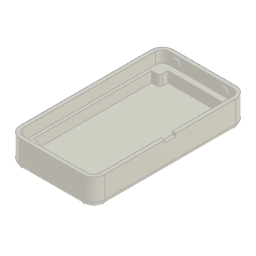
NodeMCU_Case_v9 (Autodesk Fusion 360 design; units mm, degrees)
Autodesk Fusion 360 part; units mm, degrees
note: some values were not read from the file. Set by a fixed rule: which sketch regions a step uses.
sketch "Skizze1" plane through (0, 0, 0) normal (0, 0, 1) x (1, 0, 0)
  line L0 (-15.4, 27.9) -> (15.4, 27.9)
  line L1 (15.4, 27.9) -> (15.4, -27.9)
  line L2 (15.4, -27.9) -> (-15.4, -27.9)
  line L3 (-15.4, -27.9) -> (-15.4, 27.9)
  line L4 (0, 70) -> (0, 58.2849) construction
  line L5 (30, 0) -> (40, 0) construction
  line L6 (-13.8, 26.3) -> (13.8, 26.3)
  line L7 (13.8, 26.3) -> (13.8, -26.3)
  line L8 (13.8, -26.3) -> (-13.8, -26.3)
  line L9 (-13.8, -26.3) -> (-13.8, 26.3)
  line L10 (-13, 24.5) -> (13, 24.5)
  line L11 (13, 24.5) -> (13, -24.5)
  line L12 (13, -24.5) -> (-13, -24.5)
  line L13 (-13, -24.5) -> (-13, 24.5)
  line L14 (-13, 19.5) -> (-10.03, 19.5)
  line L15 (-10.03, 19.5) -> (-10.03, -19.4987)
  line L16 (10.03, 19.5) -> (10.03, -19.4987)
  line L17 (13, 19.5) -> (10.03, 19.5)
  line L18 (-10.03, -19.4987) -> (-13, -19.4987)
  line L19 (10.03, -19.4987) -> (13, -19.4987)
  circle A0 centre (10.5, 21.7) radius 1.5
  circle A1 centre (-10.5, 21.7) radius 1.5
  circle A2 centre (10.5, -21.7) radius 1.5
  circle A3 centre (-10.5, -21.7) radius 1.5
  line L20 (-7.03, 20) -> (-7.03, -20)
  spline S0 degree 5 poles (-7.03, 20) (-6.9803, 20.007) (-6.8827, 20.0236) (-6.7413, 20.0561) (-6.5626, 20.1135) (-6.3549, 20.2028) (-6.1611, 20.3033) (-5.9792, 20.41) (-5.8066, 20.5219) (-5.6404, 20.6442) (-5.4777, 20.7847) (-5.3165, 20.9514) (-5.1557, 21.1497) (-4.9962, 21.3794) (-4.8409, 21.6328) (-4.6934, 21.8985) (-4.5577, 22.1636) (-4.4367, 22.4166) (-4.3316, 22.6498) (-4.2411, 22.8631) (-4.161, 23.0622) (-4.0871, 23.256) (-4.0155, 23.4531) (-3.9446, 23.6591) (-3.8764, 23.8734) (-3.816, 24.0904) (-3.7783, 24.2602) (-3.7581, 24.3824) (-3.7486, 24.4613) (-3.7448, 24.5) knots 0 0 0 0 0 0 0.04 0.08 0.12 0.16 0.2 0.24 0.28 0.32 0.36 0.4 0.44 0.48 0.52 0.56 0.6 0.64 0.68 0.72 0.76 0.8 0.84 0.88 0.92 0.96 1 1 1 1 1 1
  spline S1 degree 5 poles (7.03, 20) (6.9803, 20.007) (6.8827, 20.0236) (6.7413, 20.0561) (6.5626, 20.1135) (6.3549, 20.2028) (6.1611, 20.3033) (5.9792, 20.41) (5.8066, 20.5219) (5.6404, 20.6442) (5.4777, 20.7847) (5.3165, 20.9514) (5.1557, 21.1497) (4.9962, 21.3794) (4.8409, 21.6328) (4.6934, 21.8985) (4.5577, 22.1636) (4.4367, 22.4166) (4.3316, 22.6498) (4.2411, 22.8631) (4.161, 23.0622) (4.0871, 23.256) (4.0155, 23.4531) (3.9446, 23.6591) (3.8764, 23.8734) (3.816, 24.0904) (3.7783, 24.2602) (3.7581, 24.3824) (3.7486, 24.4613) (3.7448, 24.5) knots 0 0 0 0 0 0 0.04 0.08 0.12 0.16 0.2 0.24 0.28 0.32 0.36 0.4 0.44 0.48 0.52 0.56 0.6 0.64 0.68 0.72 0.76 0.8 0.84 0.88 0.92 0.96 1 1 1 1 1 1
  line L21 (-7.8289, 19.8867) -> (-6.2311, 20.1133)
  line L22 (-3.8089, 23.844) -> (-3.6806, 25.156)
  line L23 (7.8289, 19.8867) -> (6.2311, 20.1133)
  line L24 (3.8089, 23.844) -> (3.6806, 25.156)
  spline S2 degree 5 poles (-7.03, -20) (-6.9803, -20.007) (-6.8827, -20.0236) (-6.7413, -20.0561) (-6.5626, -20.1135) (-6.3549, -20.2028) (-6.1611, -20.3033) (-5.9792, -20.41) (-5.8066, -20.5219) (-5.6404, -20.6442) (-5.4777, -20.7847) (-5.3165, -20.9514) (-5.1557, -21.1497) (-4.9962, -21.3794) (-4.8409, -21.6328) (-4.6934, -21.8985) (-4.5577, -22.1636) (-4.4367, -22.4166) (-4.3316, -22.6498) (-4.2411, -22.8631) (-4.161, -23.0622) (-4.0871, -23.256) (-4.0155, -23.4531) (-3.9446, -23.6591) (-3.8764, -23.8734) (-3.816, -24.0904) (-3.7783, -24.2602) (-3.7581, -24.3824) (-3.7486, -24.4613) (-3.7448, -24.5) knots 0 0 0 0 0 0 0.04 0.08 0.12 0.16 0.2 0.24 0.28 0.32 0.36 0.4 0.44 0.48 0.52 0.56 0.6 0.64 0.68 0.72 0.76 0.8 0.84 0.88 0.92 0.96 1 1 1 1 1 1
  line L25 (-7.8289, -19.8867) -> (-6.2311, -20.1133)
  line L26 (-3.8089, -23.844) -> (-3.6806, -25.156)
  spline S3 degree 5 poles (7.03, -20) (6.9803, -20.007) (6.8827, -20.0236) (6.7413, -20.0561) (6.5626, -20.1135) (6.3549, -20.2028) (6.1611, -20.3033) (5.9792, -20.41) (5.8066, -20.5219) (5.6404, -20.6442) (5.4777, -20.7847) (5.3165, -20.9514) (5.1557, -21.1497) (4.9962, -21.3794) (4.8409, -21.6328) (4.6934, -21.8985) (4.5577, -22.1636) (4.4367, -22.4166) (4.3316, -22.6498) (4.2411, -22.8631) (4.161, -23.0622) (4.0871, -23.256) (4.0155, -23.4531) (3.9446, -23.6591) (3.8764, -23.8734) (3.816, -24.0904) (3.7783, -24.2602) (3.7581, -24.3824) (3.7486, -24.4613) (3.7448, -24.5) knots 0 0 0 0 0 0 0.04 0.08 0.12 0.16 0.2 0.24 0.28 0.32 0.36 0.4 0.44 0.48 0.52 0.56 0.6 0.64 0.68 0.72 0.76 0.8 0.84 0.88 0.92 0.96 1 1 1 1 1 1
  line L27 (7.8289, -19.8867) -> (6.2311, -20.1133)
  line L28 (3.8089, -23.844) -> (3.6806, -25.156)
  line L29 (7.03, 20) -> (7.03, -20)
  point P0 (-6, 20.4)
  point P1 (-5.2, 21.1)
  point P2 (-4.4, 22.5)
  point P3 (-4, 23.5)
  point P4 (6, 20.4)
  point P5 (5.2, 21.1)
  point P6 (4.4, 22.5)
  point P7 (4, 23.5)
  point P8 (-6, -20.4)
  point P9 (-5.2, -21.1)
  point P10 (-4.4, -22.5)
  point P11 (-4, -23.5)
  point P12 (6, -20.4)
  point P13 (5.2, -21.1)
  point P14 (4.4, -22.5)
  point P15 (4, -23.5)
  dimension "d1" = 30.8
  dimension "d2" = 55.8
  dimension "d3" = 15.4
  dimension "d4" = 27.9
  dimension "d5" = 27.6
  dimension "d6" = 52.6
  dimension "d7" = 1.6
  dimension "d8" = 1.6
  dimension "d9" = 26
  dimension "d10" = 0.8
  dimension "d11" = 49
  dimension "d12" = 1.8
  dimension "d13" = 2.97
  dimension "d15" = 19.5
  dimension "d17" = 3
  dimension "d18" = 3
  dimension "d19" = 40
  dimension "d20" = 20
  constraint horizontal L0
  constraint vertical L1
  constraint horizontal L2
  constraint vertical L3
  constraint vertical L4
  constraint horizontal L5
  constraint horizontal L6
  constraint vertical L7
  constraint horizontal L8
  constraint vertical L9
  constraint horizontal L10
  constraint vertical L11
  constraint horizontal L12
  constraint vertical L13
  constraint horizontal L14
  constraint vertical L15
  constraint symmetric L4 L14.start L17.start
  constraint symmetric L4 L14.end L16.start
  constraint symmetric L4 L15.end L16.end
  constraint coincident L13 L14.start
  constraint coincident L13 L18.end
  constraint perpendicular L13 L18
  constraint coincident L11 L19.end
  constraint perpendicular L11 L19
  constraint symmetric L4 A0 A1
  constraint symmetric L5 A0 A2
  constraint symmetric L5 A1 A3
  constraint vertical L20
  constraint coincident L10 S0.end
  constraint midpoint L20.start L21
  constraint midpoint S0.end L22
  constraint symmetric L4 L20.start S1.start
  constraint symmetric L4 P0 P4
  constraint symmetric L4 P1 P5
  constraint symmetric L4 P2 P6
  constraint symmetric L4 P3 P7
  constraint symmetric L4 S0.end S1.end
  constraint symmetric L4 L21.start L23.start
  constraint symmetric L4 L21.end L23.end
  constraint symmetric L4 L22.start L24.start
  constraint symmetric L4 L22.end L24.end
  constraint symmetric L5 L20.start L20.end
  constraint symmetric L5 P0 P8
  constraint symmetric L5 P1 P9
  constraint symmetric L5 P2 P10
  constraint symmetric L5 P3 P11
  constraint symmetric L5 S0.end S2.end
  constraint symmetric L5 S1.start S3.start
  constraint symmetric L5 P4 P12
  constraint symmetric L5 P5 P13
  constraint symmetric L5 P6 P14
  constraint symmetric L5 P7 P15
  constraint symmetric L5 S1.end S3.end
  constraint symmetric L5 L21.start L25.start
  constraint symmetric L5 L21.end L25.end
  constraint symmetric L5 L22.start L26.start
  constraint symmetric L5 L22.end L26.end
  constraint symmetric L5 L23.start L27.start
  constraint symmetric L5 L23.end L27.end
  constraint symmetric L5 L24.start L28.start
  constraint symmetric L5 L24.end L28.end
  constraint symmetric L4 L20.end S3.start
  measures "d1" distance of L0.start L0.end
  measures "d2" distance of L0.start L2.end
  measures "d3" distance of L3 L4
  measures "d4" distance of L2 L5
  measures "d5" distance of L6.start L6.end
  measures "d6" distance of L6.start L8.end
  measures "d7" distance of L0 L6
  measures "d8" distance of L3 L9
  measures "d9" distance of L10.start L10.end
  measures "d10" distance of L9 L13
  measures "d11" distance of L10.start L12.end
  measures "d12" distance of L6 L10
  measures "d13" distance of L14.start L14.end
  measures "d15" distance of L5 L14
  measures "d17" diameter of A0
  measures "d18" distance of L15 L20
  measures "d19" distance of L20.start L20.end
  measures "d20" distance of L5 L20.start
sketch "Skizze2" plane through (0, 0, 0) normal (0, 0, 1) x (1, 0, 0)
  line L0 (-7.03, 20) -> (-7.03, -20)
  line L1 (-13.8, -23.8) -> (-13.8, 23.8)
  line L2 (10.03, -19.5) -> (13, -19.5)
  line L3 (-13, -22) -> (-13, 22)
  line L4 (-10.5, 24.5) -> (10.5, 24.5)
  line L5 (-13, 19.5) -> (-10.03, 19.5)
  line L6 (-10.03, 19.5) -> (-10.03, -19.5)
  line L7 (13, 22) -> (13, -22)
  line L8 (11.3, -27.9) -> (-11.3, -27.9)
  line L9 (10.5, -24.5) -> (-10.5, -24.5)
  line L10 (-11.3, 26.3) -> (11.3, 26.3)
  line L11 (-10.03, -19.5) -> (-13, -19.5)
  line L12 (13, 19.5) -> (10.03, 19.5)
  line L13 (11.3, -26.3) -> (-11.3, -26.3)
  line L14 (-15.4, -23.8) -> (-15.4, 23.8)
  line L15 (13.8, 23.8) -> (13.8, -23.8)
  line L16 (-11.3, 27.9) -> (11.3, 27.9)
  line L17 (15.4, 23.8) -> (15.4, -23.8)
  line L18 (0, 69.9987) -> (0, 58.2836) construction
  line L19 (7.03, 20) -> (7.03, -20)
  line L20 (10.03, 19.5) -> (10.03, -19.5)
  arc A0 (-11.3, 27.9) -> (-15.4, 23.8) centre (-11.3, 23.8) ccw
  arc A1 (15.4, 23.8) -> (11.3, 27.9) centre (11.3, 23.8) ccw
  arc A2 (11.3, -27.9) -> (15.4, -23.8) centre (11.3, -23.8) ccw
  arc A3 (-15.4, -23.8) -> (-11.3, -27.9) centre (-11.3, -23.8) ccw
  arc A4 (-11.3, 26.3) -> (-13.8, 23.8) centre (-11.3, 23.8) ccw
  arc A5 (13.8, 23.8) -> (11.3, 26.3) centre (11.3, 23.8) ccw
  arc A6 (11.3, -26.3) -> (13.8, -23.8) centre (11.3, -23.8) ccw
  arc A7 (-13.8, -23.8) -> (-11.3, -26.3) centre (-11.3, -23.8) ccw
  arc A8 (-13, -22) -> (-10.5, -24.5) centre (-10.5, -22) ccw
  arc A9 (10.5, -24.5) -> (13, -22) centre (10.5, -22) ccw
  arc A10 (13, 22) -> (10.5, 24.5) centre (10.5, 22) ccw
  arc A11 (-10.5, 24.5) -> (-13, 22) centre (-10.5, 22) ccw
  line L21 (24, 0) -> (32, 0) construction
  spline S0 degree 5 poles (-7.03, -20) (-6.9979, -19.9959) (-6.9341, -19.9893) (-6.8398, -19.9844) (-6.7169, -19.9881) (-6.5682, -20.0095) (-6.4249, -20.0474) (-6.288, -20.101) (-6.159, -20.1689) (-6.0404, -20.249) (-5.9347, -20.3389) (-5.844, -20.4361) (-5.7694, -20.5386) (-5.7104, -20.6452) (-5.6648, -20.7559) (-5.6293, -20.871) (-5.6004, -20.9917) (-5.5756, -21.119) (-5.5531, -21.2541) (-5.5325, -21.3979) (-5.514, -21.5509) (-5.4979, -21.7132) (-5.4847, -21.884) (-5.4743, -22.062) (-5.4665, -22.2452) (-5.4607, -22.4315) (-5.4563, -22.6186) (-5.453, -22.8046) (-5.4501, -22.9883) (-5.4474, -23.1689) (-5.4447, -23.3461) (-5.4418, -23.5199) (-5.4387, -23.6905) (-5.4353, -23.8581) (-5.4316, -24.0228) (-5.4276, -24.1848) (-5.4241, -24.3122) (-5.4213, -24.4066) (-5.4194, -24.4689) (-5.4184, -24.5) knots 0 0 0 0 0 0 0.028571 0.057143 0.085714 0.114286 0.142857 0.171429 0.2 0.228571 0.257143 0.285714 0.314286 0.342857 0.371429 0.4 0.428571 0.457143 0.485714 0.514286 0.542857 0.571429 0.6 0.628571 0.657143 0.685714 0.714286 0.742857 0.771429 0.8 0.828571 0.857143 0.885714 0.914286 0.942857 0.971429 1 1 1 1 1 1
  spline S1 degree 5 poles (7.03, -20) (6.9979, -19.9959) (6.9341, -19.9893) (6.8398, -19.9844) (6.7169, -19.9881) (6.5682, -20.0095) (6.4249, -20.0474) (6.288, -20.101) (6.159, -20.1689) (6.0404, -20.249) (5.9347, -20.3389) (5.844, -20.4361) (5.7694, -20.5386) (5.7104, -20.6452) (5.6648, -20.7559) (5.6293, -20.871) (5.6004, -20.9917) (5.5756, -21.119) (5.5531, -21.2541) (5.5325, -21.3979) (5.514, -21.5509) (5.4979, -21.7132) (5.4847, -21.884) (5.4743, -22.062) (5.4665, -22.2452) (5.4607, -22.4315) (5.4563, -22.6186) (5.453, -22.8046) (5.4501, -22.9883) (5.4474, -23.1689) (5.4447, -23.3461) (5.4418, -23.5199) (5.4387, -23.6905) (5.4353, -23.8581) (5.4316, -24.0228) (5.4276, -24.1848) (5.4241, -24.3122) (5.4213, -24.4066) (5.4194, -24.4689) (5.4184, -24.5) knots 0 0 0 0 0 0 0.028571 0.057143 0.085714 0.114286 0.142857 0.171429 0.2 0.228571 0.257143 0.285714 0.314286 0.342857 0.371429 0.4 0.428571 0.457143 0.485714 0.514286 0.542857 0.571429 0.6 0.628571 0.657143 0.685714 0.714286 0.742857 0.771429 0.8 0.828571 0.857143 0.885714 0.914286 0.942857 0.971429 1 1 1 1 1 1
  line L22 (-7.612, -20.0749) -> (-6.448, -19.9251)
  line L23 (-5.435, -23.9731) -> (-5.4019, -25.0269)
  line L24 (7.612, -20.0749) -> (6.448, -19.9251)
  line L25 (5.435, -23.9731) -> (5.4019, -25.0269)
  spline S2 degree 5 poles (7.03, 20) (6.9979, 19.9959) (6.9341, 19.9893) (6.8398, 19.9844) (6.7169, 19.9881) (6.5682, 20.0095) (6.4249, 20.0474) (6.288, 20.101) (6.159, 20.1689) (6.0404, 20.249) (5.9347, 20.3389) (5.844, 20.4361) (5.7694, 20.5386) (5.7104, 20.6452) (5.6648, 20.7559) (5.6293, 20.871) (5.6004, 20.9917) (5.5756, 21.119) (5.5531, 21.2541) (5.5325, 21.3979) (5.514, 21.5509) (5.4979, 21.7132) (5.4847, 21.884) (5.4743, 22.062) (5.4665, 22.2452) (5.4607, 22.4315) (5.4563, 22.6186) (5.453, 22.8046) (5.4501, 22.9883) (5.4474, 23.1689) (5.4447, 23.3461) (5.4418, 23.5199) (5.4387, 23.6905) (5.4353, 23.8581) (5.4316, 24.0228) (5.4276, 24.1848) (5.4241, 24.3122) (5.4213, 24.4066) (5.4194, 24.4689) (5.4184, 24.5) knots 0 0 0 0 0 0 0.028571 0.057143 0.085714 0.114286 0.142857 0.171429 0.2 0.228571 0.257143 0.285714 0.314286 0.342857 0.371429 0.4 0.428571 0.457143 0.485714 0.514286 0.542857 0.571429 0.6 0.628571 0.657143 0.685714 0.714286 0.742857 0.771429 0.8 0.828571 0.857143 0.885714 0.914286 0.942857 0.971429 1 1 1 1 1 1
  line L26 (7.612, 20.0749) -> (6.448, 19.9251)
  line L27 (5.435, 23.9731) -> (5.4019, 25.0269)
  spline S3 degree 5 poles (-7.03, 20) (-6.9979, 19.9959) (-6.9341, 19.9893) (-6.8398, 19.9844) (-6.7169, 19.9881) (-6.5682, 20.0095) (-6.4249, 20.0474) (-6.288, 20.101) (-6.159, 20.1689) (-6.0404, 20.249) (-5.9347, 20.3389) (-5.844, 20.4361) (-5.7694, 20.5386) (-5.7104, 20.6452) (-5.6648, 20.7559) (-5.6293, 20.871) (-5.6004, 20.9917) (-5.5756, 21.119) (-5.5531, 21.2541) (-5.5325, 21.3979) (-5.514, 21.5509) (-5.4979, 21.7132) (-5.4847, 21.884) (-5.4743, 22.062) (-5.4665, 22.2452) (-5.4607, 22.4315) (-5.4563, 22.6186) (-5.453, 22.8046) (-5.4501, 22.9883) (-5.4474, 23.1689) (-5.4447, 23.3461) (-5.4418, 23.5199) (-5.4387, 23.6905) (-5.4353, 23.8581) (-5.4316, 24.0228) (-5.4276, 24.1848) (-5.4241, 24.3122) (-5.4213, 24.4066) (-5.4194, 24.4689) (-5.4184, 24.5) knots 0 0 0 0 0 0 0.028571 0.057143 0.085714 0.114286 0.142857 0.171429 0.2 0.228571 0.257143 0.285714 0.314286 0.342857 0.371429 0.4 0.428571 0.457143 0.485714 0.514286 0.542857 0.571429 0.6 0.628571 0.657143 0.685714 0.714286 0.742857 0.771429 0.8 0.828571 0.857143 0.885714 0.914286 0.942857 0.971429 1 1 1 1 1 1
  line L28 (-7.612, 20.0749) -> (-6.448, 19.9251)
  line L29 (-5.435, 23.9731) -> (-5.4019, 25.0269)
  point P0 (-13, -24.5)
  point P1 (13, 24.5)
  point P2 (-13, 24.5)
  point P3 (13.8, 26.3)
  point P4 (-13.8, -26.3)
  point P5 (-13.8, 26.3)
  point P6 (15.4, 27.9)
  point P7 (-15.4, 27.9)
  point P8 (-15.4, -27.9)
  point P9 (-6.3, -20.1)
  point P10 (-5.8, -20.5)
  point P11 (-5.6, -21)
  point P12 (-5.5, -21.7)
  point P13 (-5.4551, -22.6933)
  point P14 (-5.4391, -23.664)
  point P15 (6.3, -20.1)
  point P16 (5.8, -20.5)
  point P17 (5.6, -21)
  point P18 (5.5, -21.7)
  point P19 (5.4551, -22.6933)
  point P20 (5.4391, -23.664)
  point P21 (6.3, 20.1)
  point P22 (5.8, 20.5)
  point P23 (5.6, 21)
  point P24 (5.5, 21.7)
  point P25 (5.4551, 22.6933)
  point P26 (5.4391, 23.664)
  point P27 (-6.3, 20.1)
  point P28 (-5.8, 20.5)
  point P29 (-5.6, 21)
  point P30 (-5.5, 21.7)
  point P31 (-5.4551, 22.6933)
  point P32 (-5.4391, 23.664)
  dimension "d21" = 30.8
  dimension "d22" = 55.8
  dimension "d23" = 15.4
  dimension "d25" = 27.6
  dimension "d26" = 52.6
  dimension "d27" = 1.6
  dimension "d28" = 1.6
  dimension "d29" = 26
  dimension "d30" = 0.8
  dimension "d31" = 49
  dimension "d32" = 1.8
  dimension "d33" = 2.97
  dimension "d36" = 3
  dimension "d37" = 40
  dimension "d39" = 4.1
  dimension "d40" = 2.5
  dimension "d41" = 2.5
  dimension "d75" = 39
  dimension "d129" = 24.5
  constraint horizontal L16
  constraint vertical L17
  constraint horizontal L8
  constraint vertical L14
  constraint vertical L18
  constraint horizontal L10
  constraint vertical L15
  constraint horizontal L13
  constraint vertical L1
  constraint horizontal L4
  constraint vertical L7
  constraint horizontal L9
  constraint vertical L3
  constraint horizontal L5
  constraint vertical L6
  constraint symmetric L12.start L5.start L18
  constraint symmetric L12.end L5.end L18
  constraint symmetric L2.start L6.end L18
  constraint coincident L5.start L3
  constraint coincident L11.end L3
  constraint perpendicular L3 L11
  constraint coincident L2.end L7
  constraint perpendicular L2 L7
  constraint vertical L0
  constraint symmetric L19.start L0.start L18
  constraint symmetric L19.end L0.end L18
  constraint coincident P7 L14
  constraint coincident P7 L16
  constraint tangent L14 A0
  constraint tangent L16 A0
  constraint coincident P6 L16
  constraint coincident P6 L17
  constraint tangent L16 A1
  constraint tangent L17 A1
  constraint equal A0 A1
  constraint tangent L8 A2
  constraint tangent L17 A2
  constraint equal A0 A2
  constraint coincident P8 L8
  constraint coincident P8 L14
  constraint tangent L8 A3
  constraint tangent L14 A3
  constraint equal A0 A3
  constraint coincident P5 L1
  constraint coincident P5 L10
  constraint tangent L1 A4
  constraint tangent L10 A4
  constraint coincident P3 L10
  constraint coincident P3 L15
  constraint tangent L10 A5
  constraint tangent L15 A5
  constraint equal A4 A5
  constraint tangent L13 A6
  constraint tangent L15 A6
  constraint equal A4 A6
  constraint coincident P4 L1
  constraint coincident P4 L13
  constraint tangent L1 A7
  constraint tangent L13 A7
  constraint equal A4 A7
  constraint coincident P0 L3
  constraint coincident P0 L9
  constraint tangent L3 A8
  constraint tangent L9 A8
  constraint tangent L7 A9
  constraint tangent L9 A9
  constraint equal A8 A9
  constraint coincident P1 L4
  constraint coincident P1 L7
  constraint tangent L4 A10
  constraint tangent L7 A10
  constraint equal A8 A10
  constraint coincident P2 L3
  constraint coincident P2 L4
  constraint tangent L3 A11
  constraint tangent L4 A11
  constraint equal A8 A11
  constraint horizontal L21
  constraint coincident L9 S0.end
  constraint midpoint L0.end L22
  constraint midpoint S0.end L23
  constraint symmetric L0.end L18 L19.end
  constraint symmetric L18 P9 P15
  constraint symmetric L18 P10 P16
  constraint symmetric L18 P11 P17
  constraint symmetric L18 P12 P18
  constraint symmetric L18 P13 P19
  constraint symmetric L18 P14 P20
  constraint symmetric L18 S0.end S1.end
  constraint symmetric L18 L22.start L24.start
  constraint symmetric L18 L22.end L24.end
  constraint symmetric L18 L23.start L25.start
  constraint symmetric L18 L23.end L25.end
  constraint symmetric L0.end L21 L0.start
  constraint symmetric L21 P9 P27
  constraint symmetric L21 P10 P28
  constraint symmetric L21 P11 P29
  constraint symmetric L21 P12 P30
  constraint symmetric L21 P13 P31
  constraint symmetric L21 P14 P32
  constraint symmetric L21 S0.end S3.end
  constraint symmetric L21 L19.end L19.start
  constraint symmetric L21 P15 P21
  constraint symmetric L21 P16 P22
  constraint symmetric L21 P17 P23
  constraint symmetric L21 P18 P24
  constraint symmetric L21 P19 P25
  constraint symmetric L21 P20 P26
  constraint symmetric L21 S1.end S2.end
  constraint symmetric L21 L22.start L28.start
  constraint symmetric L21 L22.end L28.end
  constraint symmetric L21 L23.start L29.start
  constraint symmetric L21 L23.end L29.end
  constraint symmetric L21 L24.start L26.start
  constraint symmetric L21 L24.end L26.end
  constraint symmetric L21 L25.start L27.start
  constraint symmetric L21 L25.end L27.end
  measures "d21" distance of P6 P7
  measures "d22" distance of P7 P8
  measures "d23" distance of L14 L18
  measures "d25" distance of P3 P5
  measures "d26" distance of P4 P5
  measures "d27" distance of L10 L16
  measures "d28" distance of L1 L14
  measures "d29" distance of P1 P2
  measures "d30" distance of L1 L3
  measures "d31" distance of P0 P2
  measures "d32" distance of L4 L10
  measures "d33" distance of L5.end L5.start
  measures "d36" distance of L0 L6
  measures "d37" distance of L0.end L0.start
  measures "d39" radius of A0
  measures "d40" radius of A4
  measures "d41" radius of A8
  measures "d75" distance of L6.end L5.end
  measures "d129" distance of L4 L21
extrude "Extrusion1" add sketch "Skizze2" along normal blind 2 contours L0 L4 L9 L19 S0 S1 S2 S3 | L0 L3 L4 L5 L6 L9 L11 A8 A11 S0 S3 | L2 L4 L7 L9 L12 L19 L20 A9 A10 S1 S2 | L3 L5 L6 L11 | L2 L7 L12 L20 | L1 L10 L13 L15 A4 A5 A6 A7 | L8 L14 L16 L17 A0 A1 A2 A3 makes body 1
extrude "Extrusion2" add sketch "Skizze2" along normal blind 14.6 from surface at 2 contours L0 L3 L4 L5 L6 L9 L11 A8 A11 S0 S3 | L2 L4 L7 L9 L12 L19 L20 A9 A10 S1 S2 bodies 1
extrude "Extrusion3" add sketch "Skizze2" along normal blind 16.4 from surface at 2 contours L1 L10 L13 L15 A4 A5 A6 A7 bodies 1
extrude "Extrusion4" add sketch "Skizze2" along normal blind 12.4 from surface at 2 contours L8 L14 L16 L17 A0 A1 A2 A3 bodies 1
fillet "Abrundung1" radius 2 8 edges at (-14.1991, 26.6991, 0) (-15.4, 0, 0) (-14.1991, -26.6991, 0) (0, -27.9, 0) (14.1991, -26.6991, 0) (15.4, 0, 0) (14.1991, 26.6991, 0) (0, 27.9, 0) on bodies 1
sketch "Skizze3" plane through (0, -26.3, 0) normal (0, -1, 0) x (1, 0, 0)
  line L0 (-11.3, 11.4) -> (11.3, 11.4)
  line L1 (11.3, 11.4) -> (11.3, 15.4)
  line L2 (11.3, 15.4) -> (-11.3, 15.4)
  line L3 (-11.3, 15.4) -> (-11.3, 11.4)
  line L4 (0, 19.5) -> (0, 18) construction
  circle A0 centre (-8.75, 16.4) radius 1.5
  circle A1 centre (8.75, 16.4) radius 1.5
  line L5 (-11.3, 14.4) -> (11.3, 14.4)
  line L6 (11.3, 14.4) -> (11.3, 18.4)
  line L7 (11.3, 18.4) -> (-11.3, 18.4)
  line L8 (-11.3, 18.4) -> (-11.3, 14.4)
  dimension "d58" = 3
  dimension "d59" = 5
  dimension "d127" = 8.75
  constraint perpendicular L2 L4
  measures "d58" diameter of A0
  measures "d59" distance of L0 A0.centre
  measures "d127" distance of L4 A0.centre
ref_plane "Arbeitsebene4" through (0, -25.8, 14.9) normal (0, -1, 0) x (1, 0, 0)
sketch "Skizze14" plane through (0, -25.8, 13.4) normal (0, -1, 0) x (1, 0, 0)
  circle A0 centre (-8.75, 3) radius 1
  line L0 (-11.3, 1) -> (11.3, 1)
  line L1 (0, 3.5) -> (0, 2.1411) construction
  circle A1 centre (8.75, 3) radius 1
  dimension "d139" = 2
  dimension "d140" = 2
  dimension "d141" = 8.75
  constraint vertical L1
  constraint symmetric A0 L1 A1
  measures "d139" diameter of A0
  measures "d140" distance of A0.centre L0
  measures "d141" distance of A0.centre L1
sketch "Skizze12" plane through (0, 26.3, 0) normal (0, 1, 0) x (-1, 0, 0)
  line L0 (-11.3, 14.4) -> (11.3, 14.4)
  line L1 (11.3, 14.4) -> (11.3, 18.4)
  line L2 (11.3, 18.4) -> (-11.3, 18.4)
  line L3 (-11.3, 18.4) -> (-11.3, 14.4)
  circle A0 centre (-8.75, 16.4) radius 1.5
  line L4 (0, 16) -> (0, 19) construction
  circle A1 centre (8.75, 16.4) radius 1.5
  dimension "d131" = 3
  dimension "d132" = 2
  dimension "d133" = 8.75
  constraint vertical L4
  constraint symmetric A0 L4 A1
  measures "d131" diameter of A0
  measures "d132" distance of L0 A0.centre
  measures "d133" distance of A0.centre L4
ref_plane "Arbeitsebene3" through (0, 25.8, 16.4) normal (0, 1, 0) x (-1, 0, 0)
sketch "Skizze13" plane through (0, 25.8, 13.4) normal (0, 1, 0) x (1, 0, 0)
  circle A0 centre (8.75, -3) radius 1
  line L0 (11.3, -1) -> (-11.3, -1)
  line L1 (0, -2.5) -> (0, -4) construction
  circle A1 centre (-8.75, -3) radius 1
  dimension "d135" = 2
  dimension "d136" = 2
  dimension "d137" = 8.75
  constraint vertical L1
  constraint symmetric A0 L1 A1
  measures "d135" diameter of A0
  measures "d136" distance of A0.centre L0
  measures "d137" distance of A0.centre L1
loft "Erhebung5" cut profiles "Skizze14", "Skizze3" section 1 contours A0 section 2 contours L2 A0 | L2 A0 bodies 1
loft "Erhebung6" cut profiles "Skizze14", "Skizze3" section 1 contours A1 section 2 contours L2 A1 | L2 A1 bodies 1
loft "Erhebung7" cut profiles "Skizze13", "Skizze12" section 1 contours A1 section 2 contours A1 bodies 1
loft "Erhebung8" cut profiles "Skizze13", "Skizze12" section 1 contours A0 section 2 contours A0 bodies 1
sketch "Skizze8" plane through (0, 0, 18.4) normal (0, 0, 1) x (-1, 0, 0)
  line L0 (10.5, -24.5) -> (-10.5, -24.5)
  line L1 (-13, -22) -> (-13, 22)
  line L2 (-10.5, 24.5) -> (10.5, 24.5)
  line L3 (13, 22) -> (13, -22)
  line L4 (-11.3, -26.3) -> (11.3, -26.3)
  arc A0 (11.3, -26.3) -> (13.8, -23.8) centre (11.3, -23.8) ccw
  line L5 (13.8, -23.8) -> (13.8, 23.8)
  arc A1 (13.8, 23.8) -> (11.3, 26.3) centre (11.3, 23.8) ccw
  line L6 (11.3, 26.3) -> (-11.3, 26.3)
  arc A2 (-11.3, 26.3) -> (-13.8, 23.8) centre (-11.3, 23.8) ccw
  line L7 (-13.8, 23.8) -> (-13.8, -23.8)
  arc A3 (-13.8, -23.8) -> (-11.3, -26.3) centre (-11.3, -23.8) ccw
  line L8 (4.5, 24.5) -> (4.5, 26.3)
  line L9 (0, 29.5) -> (0, 28.8) construction
  line L10 (-4.5, 24.5) -> (-4.5, 26.3)
  arc A4 (-13, -22) -> (-10.5, -24.5) centre (-10.5, -22) ccw
  arc A5 (-10.5, 24.5) -> (-13, 22) centre (-10.5, 22) ccw
  arc A6 (13, 22) -> (10.5, 24.5) centre (10.5, 22) ccw
  arc A7 (10.5, -24.5) -> (13, -22) centre (10.5, -22) ccw
  dimension "d65" = 4.5
  constraint coincident L2 L8.start
  constraint coincident L6 L8.end
  constraint perpendicular L6 L8
  constraint vertical L9
  constraint symmetric L8.start L9 L10.start
  constraint symmetric L8.end L9 L10.end
  measures "d65" distance of L8 L9
extrude "Extrusion5" cut sketch "Skizze8" against normal blind 1.8 contours L2 L6 L8 L10 bodies 1
sketch "Skizze9" plane through (-7.03, 0, 0) normal (1, 0, 0) x (0, 1, 0)
  line L0 (-20, 2) -> (20, 2)
  line L1 (20, 16.6) -> (-20, 16.6)
  line L2 (-20, 9.2) -> (20, 9.2)
  line L3 (20, 2) -> (20, 16.6)
  line L4 (-20, 16.6) -> (-20, 2)
  line L5 (0, 20) -> (0, 23) construction
  dimension "d76" = 40
  dimension "d77" = 7.2
  dimension "d130" = 20
  constraint perpendicular L1 L5
  measures "d76" distance of L2.start L2.end
  measures "d77" distance of L0 L2
  measures "d130" distance of L2.end L5
extrude "Extrusion7" cut sketch "Skizze9" against normal blind 3 contours L0 L2 L3 L4 bodies 1
extrude "Extrusion8" cut sketch "Skizze9" along normal blind 17.1 contours L0 L2 L3 L4 bodies 1
sketch "Skizze10" plane through (0, 24.5, 0) normal (0, -1, 0) x (1, 0, 0)
  line L0 (-5.4184, 2) -> (5.4184, 2)
  line L1 (10.5, 18.4) -> (-10.5, 18.4)
  circle A0 centre (0, 5.1) radius 2.1
  line L2 (-5.4184, 16.6) -> (-5.4184, 2)
  line L3 (5.4184, 2) -> (5.4184, 16.6)
  line L4 (-10.5, 16.6) -> (-5.4184, 16.6)
  line L5 (5.4184, 16.6) -> (10.5, 16.6)
  line L6 (10.5, 16.6) -> (10.5, 18.4)
  line L7 (-10.5, 18.4) -> (-10.5, 16.6)
  dimension "d82" = 4.2
  dimension "d83" = 3.1
  measures "d82" diameter of A0
  measures "d83" distance of L0 A0.centre
extrude "Extrusion9" cut sketch "Skizze10" against normal blind 7 contours A0 bodies 1
fillet "Abrundung4" radius 0.75 1 edges at (-1.9579, 24.5, 5.8594) on bodies 1
sketch "Skizze11" plane through (0, 0, 0) normal (0, 0, 1) x (1, 0, 0)
  line L0 (-11.3, 27.9) -> (11.3, 27.9)
  line L1 (15.4, 23.8) -> (15.4, -23.8)
  line L2 (11.3, -27.9) -> (-11.3, -27.9)
  line L3 (-15.4, -23.8) -> (-15.4, 23.8)
  line L4 (26, 0) -> (39, 0) construction
  line L5 (0, 51) -> (0, 44) construction
  line L6 (-11.6, 26.6) -> (11.6, 26.6)
  line L7 (14.1, 24.1) -> (14.1, -24.1)
  line L8 (11.6, -26.6) -> (-11.6, -26.6)
  line L9 (-14.1, -24.1) -> (-14.1, 24.1)
  line L10 (-10.5, 24.5) -> (10.5, 24.5)
  line L11 (13, 22) -> (13, -22)
  line L12 (10.5, -24.5) -> (-10.5, -24.5)
  line L13 (-13, -22) -> (-13, 22)
  arc A0 (-11.3, 27.9) -> (-15.4, 23.8) centre (-11.3, 23.8) ccw
  arc A1 (15.4, 23.8) -> (11.3, 27.9) centre (11.3, 23.8) ccw
  arc A2 (11.3, -27.9) -> (15.4, -23.8) centre (11.3, -23.8) ccw
  arc A3 (-15.4, -23.8) -> (-11.3, -27.9) centre (-11.3, -23.8) ccw
  arc A4 (-11.6, 26.6) -> (-14.1, 24.1) centre (-11.6, 24.1) ccw
  arc A5 (14.1, 24.1) -> (11.6, 26.6) centre (11.6, 24.1) ccw
  arc A6 (11.6, -26.6) -> (14.1, -24.1) centre (11.6, -24.1) ccw
  arc A7 (-14.1, -24.1) -> (-11.6, -26.6) centre (-11.6, -24.1) ccw
  arc A8 (-13, -22) -> (-10.5, -24.5) centre (-10.5, -22) ccw
  arc A9 (10.5, -24.5) -> (13, -22) centre (10.5, -22) ccw
  arc A10 (13, 22) -> (10.5, 24.5) centre (10.5, 22) ccw
  arc A11 (-10.5, 24.5) -> (-13, 22) centre (-10.5, 22) ccw
  circle A12 centre (6.15, -21.2) radius 1.5
  line L14 (0, -32) -> (0, -35) construction
  circle A13 centre (-6.15, -21.2) radius 1.5
  line L15 (-10, 24.5) -> (-10, 22.5)
  line L16 (-11, 21.5) -> (-13, 21.5)
  arc A14 (-11, 21.5) -> (-10, 22.5) centre (-11, 22.5) ccw
  line L17 (11, 21.5) -> (13, 21.5)
  arc A15 (10, 22.5) -> (11, 21.5) centre (11, 22.5) ccw
  line L18 (10, 24.5) -> (10, 22.5)
  line L19 (11, -21.5) -> (13, -21.5)
  arc A16 (11, -21.5) -> (10, -22.5) centre (11, -22.5) ccw
  line L20 (10, -24.5) -> (10, -22.5)
  line L21 (-11, -21.5) -> (-13, -21.5)
  arc A17 (-10, -22.5) -> (-11, -21.5) centre (-11, -22.5) ccw
  line L22 (-10, -24.5) -> (-10, -22.5)
  point P0 (-15.4, 27.9)
  point P1 (15.4, 27.9)
  point P2 (-15.4, -27.9)
  point P3 (-14.1, 26.6)
  point P4 (14.1, 26.6)
  point P5 (-14.1, -26.6)
  point P6 (-13, 24.5)
  point P7 (13, 24.5)
  point P8 (-13, -24.5)
  point P9 (-10, 21.5)
  dimension "d14" = 39
  dimension "d90" = 55.8
  dimension "d91" = 30.8
  dimension "d92" = 15.4
  dimension "d93" = 27.9
  dimension "d94" = 28.2
  dimension "d95" = 53.2
  dimension "d96" = 26.6
  dimension "d97" = 14.1
  dimension "d98" = 26
  dimension "d99" = 49
  dimension "d100" = 13
  dimension "d101" = 24.5
  dimension "d102" = 4.1
  dimension "d103" = 2.5
  dimension "d104" = 2.5
  dimension "d105" = 3
  dimension "d106" = 3.3
  dimension "d107" = 6.85
  dimension "d116" = 3
  dimension "d117" = 3
  dimension "d118" = 3
  dimension "d119" = 1
  constraint horizontal L0
  constraint vertical L1
  constraint horizontal L2
  constraint vertical L3
  constraint horizontal L4
  constraint vertical L5
  constraint horizontal L6
  constraint vertical L7
  constraint horizontal L8
  constraint vertical L9
  constraint horizontal L10
  constraint vertical L11
  constraint horizontal L12
  constraint vertical L13
  constraint coincident P0 L0
  constraint coincident P0 L3
  constraint tangent L0 A0
  constraint tangent L3 A0
  constraint coincident P1 L0
  constraint coincident P1 L1
  constraint tangent L0 A1
  constraint tangent L1 A1
  constraint equal A0 A1
  constraint tangent L1 A2
  constraint tangent L2 A2
  constraint equal A0 A2
  constraint coincident P2 L2
  constraint coincident P2 L3
  constraint tangent L2 A3
  constraint tangent L3 A3
  constraint equal A0 A3
  constraint coincident P3 L6
  constraint coincident P3 L9
  constraint tangent L6 A4
  constraint tangent L9 A4
  constraint coincident P4 L6
  constraint coincident P4 L7
  constraint tangent L6 A5
  constraint tangent L7 A5
  constraint equal A4 A5
  constraint tangent L7 A6
  constraint tangent L8 A6
  constraint equal A4 A6
  constraint coincident P5 L8
  constraint coincident P5 L9
  constraint tangent L8 A7
  constraint tangent L9 A7
  constraint equal A4 A7
  constraint coincident P8 L12
  constraint coincident P8 L13
  constraint tangent L12 A8
  constraint tangent L13 A8
  constraint tangent L11 A9
  constraint tangent L12 A9
  constraint equal A8 A9
  constraint coincident P7 L10
  constraint coincident P7 L11
  constraint tangent L10 A10
  constraint tangent L11 A10
  constraint equal A8 A10
  constraint coincident P6 L10
  constraint coincident P6 L13
  constraint tangent L10 A11
  constraint tangent L13 A11
  constraint equal A8 A11
  constraint perpendicular L12 L14
  constraint symmetric A12 L14 A13
  constraint coincident L10 L15.start
  constraint perpendicular L10 L15
  constraint perpendicular L13 L16
  constraint coincident P9 L15
  constraint coincident P9 L16
  constraint tangent L15 A14
  constraint tangent L16 A14
  constraint symmetric L14 L15.start L18.start
  constraint symmetric L14 L16.end L17.end
  constraint symmetric L14 L15.end A15.start
  constraint symmetric L14 L16.start L17.start
  constraint symmetric L14 A14 A15
  constraint symmetric L4 L15.start L22.start
  constraint symmetric L4 L16.end L21.end
  constraint symmetric L4 L15.end A17.start
  constraint symmetric L4 L16.start L21.start
  constraint symmetric L4 A14 A17
  constraint symmetric L4 L17.start L19.start
  constraint symmetric L4 L17.end L19.end
  constraint symmetric L4 A15.start A16.end
  constraint symmetric L4 A15 A16
  constraint symmetric L4 L18.start L20.start
  measures "d90" distance of P0 P2
  measures "d91" distance of P0 P1
  measures "d92" distance of L3 L5
  measures "d93" distance of L2 L4
  measures "d94" distance of P3 P4
  measures "d95" distance of P3 P5
  measures "d96" distance of L4 L8
  measures "d97" distance of L5 L9
  measures "d98" distance of P6 P7
  measures "d99" distance of P6 P8
  measures "d100" distance of L5 L13
  measures "d101" distance of L4 L12
  measures "d102" radius of A0
  measures "d103" radius of A4
  measures "d104" radius of A8
  measures "d105" diameter of A12
  measures "d106" distance of L12 A12.centre
  measures "d107" distance of L11 A12.centre
  measures "d116" distance of L15.start P9
  measures "d117" distance of P9 L16.end
  measures "d118" distance of L13 L15
  measures "d119" radius of A14
extrude "Extrusion10" add sketch "Skizze11" along normal blind 2 separate body contours L0 L1 L2 L3 A0 A1 A2 A3 | L6 L7 L8 L9 A4 A5 A6 A7 | L10 L13 A11 L15 L16 A14 | L10 L11 L12 L13 L15 L16 A14 L17 A15 L18 L19 A16 L20 L21 A17 L22 | L10 L11 A10 L17 A15 L18 | L12 L13 A8 L21 A17 L22 | L11 L12 A9 L19 A16 L20 makes body 2
extrude "Extrusion11" add sketch "Skizze11" along normal blind 3.8 from surface at 2 contours L6 L7 L8 L9 A4 A5 A6 A7 bodies 2
extrude "Extrusion12" add sketch "Skizze11" along normal blind 8 from surface at 2 contours L0 L1 L2 L3 A0 A1 A2 A3 bodies 2
extrude "Extrusion13" add sketch "Skizze11" along normal blind 3.8 from surface at 2 contours L10 L13 A11 L15 L16 A14 | L10 L11 A10 L17 A15 L18 | L12 L13 A8 L21 A17 L22 | L11 L12 A9 L19 A16 L20 bodies 2
fillet "Abrundung5" radius 1.5 2 edges at (4.7515, -20.6576, 0) (-7.5485, -20.6576, 0) on bodies 2
fillet "Abrundung6" radius 2 8 edges at (14.1991, 26.6991, 0) (0, 27.9, 0) (-14.1991, 26.6991, 0) (-15.4, 0, 0) (-14.1991, -26.6991, 0) (0, -27.9, 0) (14.1991, -26.6991, 0) (15.4, 0, 0) on bodies 2
sketch "Skizze15" plane through (0, 26.6, 0) normal (0, -1, 0) x (1, 0, 0)
  line L0 (-11.6, 5.8) -> (11.6, 5.8)
  line L1 (11.6, 5.8) -> (11.6, 10)
  line L2 (11.6, 10) -> (-11.6, 10)
  line L3 (-11.6, 10) -> (-11.6, 5.8)
  circle A0 centre (-8.75, 8) radius 1.5
  line L4 (0, 14) -> (0, 12) construction
  circle A1 centre (8.75, 8) radius 1.5
  dimension "d142" = 3
  dimension "d143" = 8.75
  dimension "d144" = 2.2
  constraint vertical L4
  constraint symmetric A0 L4 A1
  measures "d142" diameter of A0
  measures "d143" distance of A0.centre L4
  measures "d144" distance of L0 A0.centre
ref_plane "Arbeitsebene5" through (0, 26.1, 7.9) normal (0, -1, 0) x (1, 0, 0)
sketch "Skizze16" plane through (0, 26.1, 7.9) normal (0, -1, 0) x (1, 0, 0)
  circle A0 centre (-8.75, 0.1) radius 1
  line L0 (0, 6.5) -> (0, 4.5) construction
  line L1 (11.6, -2.1) -> (-11.6, -2.1)
  circle A1 centre (8.75, 0.1) radius 1
  dimension "d146" = 2
  dimension "d147" = 8.75
  dimension "d148" = 2.2
  constraint vertical L0
  constraint symmetric A0 L0 A1
  measures "d146" diameter of A0
  measures "d147" distance of A0.centre L0
  measures "d148" distance of A0.centre L1
sketch "Skizze17" plane through (0, -26.6, 0) normal (0, 1, 0) x (-1, 0, 0)
  line L0 (-11.6, 5.8) -> (11.6, 5.8)
  line L1 (11.6, 5.8) -> (11.6, 10)
  line L2 (11.6, 10) -> (-11.6, 10)
  line L3 (-11.6, 10) -> (-11.6, 5.8)
  circle A0 centre (-8.75, 8) radius 1.5
  line L4 (0, 14.5) -> (0, 13) construction
  circle A1 centre (8.75, 8) radius 1.5
  dimension "d149" = 3
  dimension "d150" = 8.75
  dimension "d151" = 2.2
  constraint vertical L4
  constraint symmetric A0 L4 A1
  measures "d149" diameter of A0
  measures "d150" distance of A0.centre L4
  measures "d151" distance of L0 A0.centre
ref_plane "Arbeitsebene6" through (0, -26.1, 7.9) normal (0, 1, 0) x (-1, 0, 0)
sketch "Skizze18" plane through (0, -26.1, 7.9) normal (0, 1, 0) x (1, 0, 0)
  circle A0 centre (8.75, -0.1) radius 1
  line L0 (0, -10) -> (0, -3) construction
  line L1 (11.6, 2.1) -> (-11.6, 2.1)
  circle A1 centre (-8.75, -0.1) radius 1
  dimension "d153" = 2
  dimension "d154" = 8.75
  dimension "d155" = 2.2
  constraint vertical L0
  constraint symmetric A0 L0 A1
  measures "d153" diameter of A0
  measures "d154" distance of A0.centre L0
  measures "d155" distance of A0.centre L1
loft "Erhebung9" add profiles "Skizze17", "Skizze18" section 1 contours A1 section 2 contours A1 bodies 2
loft "Erhebung10" add profiles "Skizze17", "Skizze18" section 1 contours A0 section 2 contours A0 bodies 2
loft "Erhebung11" add profiles "Skizze15", "Skizze16" section 1 contours A1 section 2 contours A1 bodies 2
loft "Erhebung12" add profiles "Skizze15", "Skizze16" section 1 contours A0 section 2 contours A0 bodies 2
fillet "Abrundung7" radius 1 1 edges at (-1.9579, 27.9, 4.3406) on bodies 1
sketch "Skizze19" plane through (0, 0, 5.8) normal (0, 0, 1) x (-1, 0, 0)
  line L0 (10, -24.5) -> (-10, -24.5)
  line L1 (-10, -24.5) -> (-10, -22.5)
  arc A0 (-10, -22.5) -> (-11, -21.5) centre (-11, -22.5) ccw
  line L2 (-11, -21.5) -> (-13, -21.5)
  line L3 (-13, -21.5) -> (-13, 21.5)
  line L4 (-13, 21.5) -> (-11, 21.5)
  arc A1 (-11, 21.5) -> (-10, 22.5) centre (-11, 22.5) ccw
  line L5 (-10, 22.5) -> (-10, 24.5)
  line L6 (-10, 24.5) -> (10, 24.5)
  line L7 (10, 24.5) -> (10, 22.5)
  arc A2 (10, 22.5) -> (11, 21.5) centre (11, 22.5) ccw
  line L8 (11, 21.5) -> (13, 21.5)
  line L9 (13, 21.5) -> (13, -21.5)
  line L10 (13, -21.5) -> (11, -21.5)
  arc A3 (11, -21.5) -> (10, -22.5) centre (11, -22.5) ccw
  line L11 (10, -22.5) -> (10, -24.5)
  line L12 (-11.6, -26.6) -> (11.6, -26.6)
  arc A4 (11.6, -26.6) -> (14.1, -24.1) centre (11.6, -24.1) ccw
  line L13 (14.1, -24.1) -> (14.1, 24.1)
  arc A5 (14.1, 24.1) -> (11.6, 26.6) centre (11.6, 24.1) ccw
  line L14 (11.6, 26.6) -> (-11.6, 26.6)
  arc A6 (-11.6, 26.6) -> (-14.1, 24.1) centre (-11.6, 24.1) ccw
  line L15 (-14.1, 24.1) -> (-14.1, -24.1)
  arc A7 (-14.1, -24.1) -> (-11.6, -26.6) centre (-11.6, -24.1) ccw
  line L16 (4.5, 24.5) -> (4.5, 26.6)
  line L17 (0, 21) -> (0, 22) construction
  line L18 (-4.5, 24.5) -> (-4.5, 26.6)
  dimension "d158" = 4.5
  constraint coincident L6 L16.start
  constraint coincident L14 L16.end
  constraint perpendicular L14 L16
  constraint vertical L17
  constraint symmetric L16.start L17 L18.start
  constraint symmetric L16.end L17 L18.end
  measures "d158" distance of L16 L17
extrude "Extrusion14" cut sketch "Skizze19" against normal blind 3.8 contours L6 L14 L16 L18 bodies 2
sketch "Skizze20" plane through (15.4, 0, 0) normal (1, 0, 0) x (0, 1, 0)
  line L0 (-23.8, 2) -> (23.8, 2)
  line L1 (23.8, 2) -> (23.8, 10)
  line L2 (23.8, 10) -> (-23.8, 10)
  line L3 (-23.8, 10) -> (-23.8, 2)
  line L4 (-2, 10) -> (-2, 9)
  line L5 (0, 12.5) -> (0, 11.5) construction
  line L6 (2, 10) -> (2, 9)
  line L7 (-2, 9) -> (2, 9)
  dimension "d161" = 1
  dimension "d162" = 2
  constraint coincident L2 L4.start
  constraint perpendicular L2 L4
  constraint vertical L5
  constraint symmetric L4.start L5 L6.start
  constraint symmetric L4.end L5 L6.end
  measures "d161" distance of L4.start L4.end
  measures "d162" distance of L4 L5
extrude "Extrusion15" cut sketch "Skizze20" against normal blind 2.5 contours L2 L4 L6 L7 bodies 2
hidden bodies 1
equation "d3 = d1 / 2"
equation "d4 = d2 / 2"
equation "d5 = d1 - ( 2 * 1.6 ) * 1 mm"
equation "d6 = d2 - ( 2 * 1.6 ) * 1 mm"
equation "d7 = ( d1 - d5 ) / 2"
equation "d8 = ( d1 - d5 ) / 2"
equation "d9 = d5 - ( 2 * 0.8 ) * 1 mm"
equation "d10 = ( d5 - d9 ) / 2"
equation "d11 = d6 - ( 2 * 1.8 ) * 1 mm"
equation "d12 = ( d6 - d11 ) / 2"
equation "d15 = d14 / 2"
equation "d20 = d19 / 2"
equation "d23 = d1 / 2"
equation "d25 = d1 - ( 2 * 1.6 ) * 1 mm"
equation "d26 = d2 - ( 2 * 1.6 ) * 1 mm"
equation "d27 = ( d1 - d5 ) / 2"
equation "d28 = ( d1 - d5 ) / 2"
equation "d29 = d5 - ( 2 * 0.8 ) * 1 mm"
equation "d30 = ( d5 - d9 ) / 2"
equation "d31 = d6 - ( 2 * 1.8 ) * 1 mm"
equation "d32 = ( d6 - d11 ) / 2"
equation "d48 = 14.6 mm + 1.8 mm"
equation "d51 = 14.6 mm + 1.8 mm - 4 mm"
equation "d83 = d82 / 2 + 1 mm"
equation "d92 = d91 / 2"
equation "d93 = d90 / 2"
equation "d96 = d95 / 2"
equation "d97 = d94 / 2"
equation "d100 = d98 / 2"
equation "d101 = d99 / 2"
equation "d129 = d31 / 2"
equation "d130 = d76 / 2"
named bodies: "Gehäuse_Bottom", "Gehäuse_Top"
